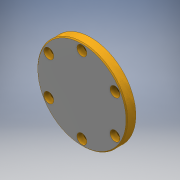
# Autodesk Inventor part: Крышка большая_72
Saved by Autodesk Inventor 2016 (Build 200138000, 138)
## iProperties
Created: 2021-04-23
Part Number: Крышка большая_72
Material: Типовые
Document SubType Name: Modeling
Designer: Лол
Density: 1 g/cm^3
Appearance: Сварка — латунь
Author: Лол
Autodesk Inventor part; units mm, degrees
ref_plane "YZ Plane" through (0, 0, 0) normal (1, 0, 0) x (0, 1, 0)
ref_plane "XZ Plane" through (0, 0, 0) normal (0, 1, 0) x (-1, 0, 0)
ref_plane "XY Plane" through (0, 0, 0) normal (0, 0, 1) x (1, 0, 0)
sketch "Эскиз1" plane through (0, 0, 0) normal (0, 0, 1) x (1, 0, 0)
  line L0 (0, 5) -> (0, 0)
  line L1 (0, 0) -> (36, 0)
  line L2 (36, 0) -> (36, 20)
  line L3 (36, 20) -> (31, 20)
  line L4 (31, 20) -> (31, 5)
  line L5 (31, 5) -> (0, 5)
  dimension "d0" = 5
  dimension "d1" = 5
  dimension "d3" = 20
  dimension "d4" = 36
  constraints: 12 end point, 4 perpendicular, 1 parallel, 1 vertical
  measures "d0" distance of L0.start L0.end
  measures "d1" distance of L2.end L3.end
  measures "d3" distance of L1.end L2.end
  measures "d4" distance of L0.end L1.end
revolve "Вращение1" add sketch "Эскиз1" angle 360 about axis through (0, 5, 0) along (0, -1, 0)
sketch "Эскиз2" plane through (0, 0, 0) normal (1, 0, 0) x (0, 1, 0)
  line L0 (-4, 0) -> (24, 0) projected
  line L1 (0, -50.4) -> (0, 50.4) projected
  line L2 (0, 0) -> (0, 50)
  line L3 (0, 50) -> (10, 50)
  line L4 (10, 50) -> (10, 0)
  line L5 (0, 0) -> (10, 0)
  line L6 (20, 36) -> (0, 36) projected
  dimension "d6" = 10
  dimension "d7" = 50
  constraints: 8 end point, 2 point on line, 1 horizontal, 1 midpoint
  measures "d6" distance of L2.end L3.end
  measures "d7" distance between parallel lines of L3 L0
revolve "Вращение2" add sketch "Эскиз2" angle 360 about axis through (0, -10, 0) along (0, 1, 0)
chamfer "Фаска1" distance 1 angle 45 1 edges at (0, 0, -50)
sketch "Эскиз3" plane through (0, 0, 0) normal (0, -1, 0) x (1, 0, 0)
  circle A0 centre (0, 0) radius 42.5 construction
  circle A1 centre (0, 42.5) radius 5.5
  line L0 (0, -70) -> (0, 70) projected
  line L1 (-70, 0) -> (70, 0) projected
  dimension "d10" = 85
  dimension "d9" = 11
  constraints: 2 coincident, 1 centre point, 1 point on line, 1 vertical alignment, 2 other
  measures "d9" diameter of A1
hole "Отверстие1" at (0, 0, 42.5) direction (0, 1, 0) diameter 6.2 depth 15 tip angle 118 counterbore diameter 11 counterbore depth 6.8
pattern_circular "Круговой массив1" count 6 over 360 about axis through (0, -10, 0) along (0, 1, 0) of "Отверстие1"
sketch "Эскиз4" plane through (0, 20, 0) normal (0, 1, 0) x (1, 0, 0)
  circle A0 centre (0, 0) radius 36 projected
  circle A1 centre (0, 0) radius 31 projected
  circle A2 centre (0, 0) radius 31
  circle A3 centre (0, 0) radius 36
  dimension "d27" = 72
  constraints: 2 centre point, 2 coincident, 1 concentric
  measures "d27" diameter of A3
extrude "Выдавливание2" add sketch "Эскиз4" along normal blind 1
fillet "Сопряжение1" radius 1.3 1 edges at (-36, 10, 0)
sketch "Эскиз5" plane through (0, 21, 0) normal (0, 1, 0) x (1, 0, 0)
  circle A0 centre (0, 0) radius 31 projected
  circle A1 centre (0, 0) radius 36 projected
  point P0 (0, 0)
extrude "Выдавливание3" cut sketch "Эскиз5" against normal blind 3
chamfer "Фаска2" distance 2 angle 45 1 edges at (-36, 18, 0)
